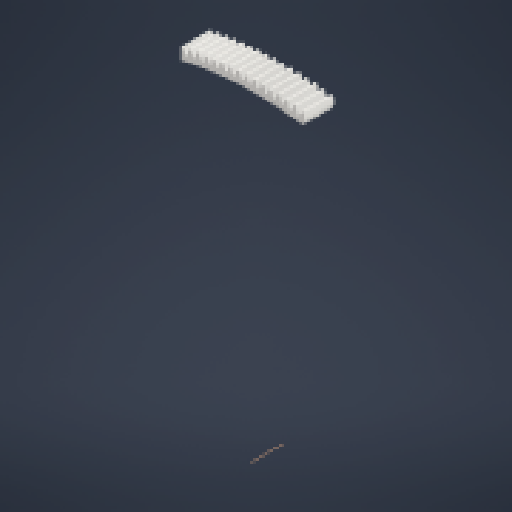
# Autodesk Inventor part: Цилиндрическое зубчатое зацепление2
Saved by Autodesk Inventor 2026.2 (Build 302298000, 298)
## iProperties
CustomPartVersion: 1
Created: 2025-12-07
Part Number: Цилиндрическое зубчатое зацепление2
Material: Steel
Document SubType Name: Modeling
Designer: Phantom
Categories: <?xml version="1.0" encoding="UTF-16"?> <MemberInstance><Categories><FamilyTemplate><FamilyTemplateParameter ValueType="xs:double" Id="1" ObjectReferenceKey="da_z" ObjectType="kUserParameterObject"/><FamilyTemplateParameter ValueType="xs:double" Id="2" ObjectReferenceKey="da_b" ObjectType="kUserParameterObject"/><FamilyTemplateParameter ValueType="xs:double" Id="3" ObjectReferenceKey="da_beta" ObjectType="kUserParameterObject"/><FamilyTemplateParameter ValueType="xs:double" Id="4" ObjectReferenceKey="da_da" ObjectType="kUserParameterObject"/><FamilyTemplateParameter ValueType="xs:double" Id="5" ObjectReferenceKey="da_aw" ObjectType="kUserParameterObject"/><FamilyTemplateParameter ValueType="xs:string" Id="6" ObjectReferenceKey="EAIAABAAAACIAQAAAAAAAIAAAAAAAAAA" ObjectType="83910656" SubObjectId="SurfaceGeometry"/></FamilyTemplate><ParamToTemplateMap><ParamToTemplate CategoryParameter="//CategoryParameter[@InternalName='046C89C9-8512-4d59-83FE-43B91F4F132A']" TemplateParameter="1"/><ParamToTemplate CategoryParameter="//CategoryParameter[@InternalName='2552DF32-E462-4b46-AEBF-C6C7768E72AC']" TemplateParameter="2"/><ParamToTemplate CategoryParameter="//CategoryParameter[@InternalName='C9EE641D-15FC-4fae-A226-E94C4372FDD7']" TemplateParameter="3"/><ParamToTemplate><ParamToTemplate CategoryParameter="//CategoryParameter[@InternalName='00B6519A-459B-49c7-AD84-2E56D39A5744']" ConstantValue="0.580360"/></ParamToTemplate><ParamToTemplate><ParamToTemplate CategoryParameter="//CategoryParameter[@InternalName='04B31F0E-C7A6-4894-AA32-9629BEFACF47']" ConstantValue="1.000000"/></ParamToTemplate><ParamToTemplate><ParamToTemplate CategoryParameter="//CategoryParameter[@InternalName='43CBEC2E-7847-49e7-A936-2F7889FCB2D9']" ConstantValue="0.250000"/></ParamToTemplate><ParamToTemplate><ParamToTemplate CategoryParameter="//CategoryParameter[@InternalName='B1EFC894-105D-4ebd-86BF-FA20ED196853']" ConstantValue="0.350000"/></ParamToTemplate><ParamToTemplate><ParamToTemplate CategoryParameter="//CategoryParameter[@InternalName='51175063-3D10-4879-93E8-6246FE8B403D']" ConstantValue="2060000000.000000"/></ParamToTemplate><ParamToTemplate><ParamToTemplate CategoryParameter="//CategoryParameter[@InternalName='A3A52E27-4454-46a9-B0BD-C932399B70AF']" ConstantValue="0.300000"/></ParamToTemplate><ParamToTemplate><ParamToTemplate CategoryParameter="//CategoryParameter[@InternalName='91B76062-C214-41d9-B1B9-14D2AB99603D']" ConstantValue="0.175000"/></ParamToTemplate><ParamToTemplate><ParamToTemplate CategoryParameter="//CategoryParameter[@InternalName='374E806E-8B8A-4dda-A9AA-1039D6500AD2']" ConstantValue="5.714286"/></ParamToTemplate><ParamToTemplate><ParamToTemplate CategoryParameter="//CategoryParameter[@InternalName='2D373A89-B862-43d6-8D0B-0CBF12AB9F6C']" ConstantValue="0.349066"/></ParamToTemplate><ParamToTemplate CategoryParameter="//CategoryParameter[@InternalName='37777632-D6A2-4fac-9D53-DB8ACD95C989']" TemplateParameter="4"/><ParamToTemplate CategoryParameter="//CategoryParameter[@InternalName='FD1017F1-B727-4f7e-9707-0F86F1FF9423']" TemplateParameter="5"/><ParamToTemplate><ParamToTemplate CategoryParameter="//CategoryParameter[@InternalName='9E1B4470-B2D3-4ff1-B813-535BB4CDF51A']" ConstantValue="3520000.000000"/></ParamToTemplate><ParamToTemplate><ParamToTemplate CategoryParameter="//CategoryParameter[@InternalName='F8452263-BFF6-458c-9FB1-07C4B99E95CD']" ConstantValue="11400000.000000"/></ParamToTemplate><ParamToTemplate><ParamToTemplate CategoryParameter="//CategoryParameter[@InternalName='3E3BB259-FD49-497f-8171-6EBC954A3479']" ConstantValue="2.000000"/></ParamToTemplate><ParamToTemplate CategoryParameter="//CategoryParameter[@InternalName='27C3BAF2-7550-4e4b-AE2C-0DB134B7D9B7']" TemplateParameter="6"/></ParamToTemplateMap><Category DisplayName="Gear" InternalName="DC85795E-93AB-48d5-8EEE-5A27447B64BD" Mnemonic="Gear"><CategoryParameter DisplayName="z" InternalName="046C89C9-8512-4d59-83FE-43B91F4F132A" Mnemonic="z"/><CategoryParameter DisplayName="b" InternalName="2552DF32-E462-4b46-AEBF-C6C7768E72AC" Mnemonic="b"/><CategoryParameter DisplayName="||b|" InternalName="C9EE641D-15FC-4fae-A226-E94C4372FDD7" Mnemonic="beta"/><CategoryParameter DisplayName="x" InternalName="00B6519A-459B-49c7-AD84-2E56D39A5744" Mnemonic="x"/><CategoryParameter DisplayName="a*" InternalName="04B31F0E-C7A6-4894-AA32-9629BEFACF47" Mnemonic="a"/><CategoryParameter DisplayName="c*" InternalName="43CBEC2E-7847-49e7-A936-2F7889FCB2D9" Mnemonic="c"/><CategoryParameter DisplayName="r|.f|*" InternalName="B1EFC894-105D-4ebd-86BF-FA20ED196853" Mnemonic="rf"/><CategoryParameter DisplayName="E" InternalName="51175063-3D10-4879-93E8-6246FE8B403D" Mnemonic="E"/><CategoryParameter DisplayName="||m|" InternalName="A3A52E27-4454-46a9-B0BD-C932399B70AF" Mnemonic="mi"/><Category DisplayName="SpurGear" InternalName="26C5A22E-A91E-4dfd-A3B3-23CCAFAE1764" Mnemonic="SpurGear"><CategoryParameter DisplayName="m" InternalName="91B76062-C214-41d9-B1B9-14D2AB99603D" Mnemonic="m"/><CategoryParameter DisplayName="P" InternalName="374E806E-8B8A-4dda-A9AA-1039D6500AD2" Mnemonic="PP"/><CategoryParameter DisplayName="||a|" InternalName="2D373A89-B862-43d6-8D0B-0CBF12AB9F6C" Mnemonic="alpha"/><CategoryParameter DisplayName="d|.a|" InternalName="37777632-D6A2-4fac-9D53-DB8ACD95C989" Mnemonic="da"/><CategoryParameter DisplayName="a|.w|" InternalName="FD1017F1-B727-4f7e-9707-0F86F1FF9423" Mnemonic="aw"/><CategoryParameter DisplayName="||s||.Flim|" InternalName="9E1B4470-B2D3-4ff1-B813-535BB4CDF51A" Mnemonic="sFlim"/><CategoryParameter DisplayName="||s||.Hlim|" InternalName="F8452263-BFF6-458c-9FB1-07C4B99E95CD" Mnemonic="sHlim"/><CategoryParameter DisplayName="тип" InternalName="3E3BB259-FD49-497f-8171-6EBC954A3479" Mnemonic="type"/><CategoryParameter DisplayName="PitchDiameter" InternalName="27C3BAF2-7550-4e4b-AE2C-0DB134B7D9B7" Mnemonic="IDS_PITCHDIAM"/></Category></Category></Categories></MemberInstance>
Density: 1 g/cm^3
Appearance: Steel
Author: Phantom
Autodesk Inventor part; units mm, degrees
sketch "Sketch1" plane through (0, 0, 0) normal (0, 0, 1) x (1, 0, 0)
  circle A0 centre (0, 0) radius 225.875
  dimension "d0" = 451.75
  constraints: 1 centre point
  measures "d0" diameter of A0
extrude "Extrusion1" add sketch "Sketch1" along normal blind 20
ref_plane "Work Plane2" through (0, 0, 10) normal (0, 0, 1) x (1, 0, 0)
sketch "Sketch2" plane through (0, 0, 0) normal (0, 0, -1) x (-1, 0, 0)
  circle A0 centre (0, 0) radius 225.875 projected
  circle A1 centre (0, 0) radius 223.125
  dimension "d3" = 446.25
  constraints: 1 centre point, 1 coincident
  measures "d3" diameter of A1
surface extrude "Средний диаметр" sketch "Sketch2" against normal through all shown no curves A1
ref_plane "Work Plane8" through (0, 0, 0) normal (0.9999241, 0.0123197, 0) x (0, 0, 1)
ref_plane "Work Plane9" through (0, 0, 0) normal (1, 0, 0) x (0, 1, 0)
spur gear teeth "Цилиндрическое зубчатое зацепление" teeth 255 pitch diameter 446.25 tip diameter 451.75 root diameter 443.9063 face width 20 start plane through (0, 0, 0) normal (0, 0, -1) x (-1, 0, 0)
sketch "Эскиз3" plane through (0, 0, 20) normal (0, 0, 1) x (1, 0, 0)
  line L0 (-50.0802, 214.6531) -> (-50.0464, 212.2194) projected
  line L1 (35.7305, 217.5025) -> (34.832, 215.2404) projected
  line L2 (-50.0802, 214.6531) -> (-50.0802, 276.5241)
  line L3 (34.832, 215.2404) -> (59.7862, 278.0604)
  line L4 (35.7305, 217.5025) -> (36.2471, 218.803) projected
  circle A0 centre (0, 0) radius 218.0406
  circle A1 centre (0, 0) radius 281.0224
  point P0 (58.5159, 274.8626)
  constraints: 4 end point, 2 coincident, 1 collinear, 1 vertical, 6 other
extrude "Выдавливание2" cut sketch "Эскиз3" against normal through all contours L0 A0 L1 L3 A1 L2 | A0 picked at (-244.7051, -87.2795)
sketch "Эскиз4" plane through (0, 0, 0) normal (0, 0, -1) x (-1, 0, 0)
  line L0 (50.0802, 214.6531) -> (50.0802, 220.2532) projected
  arc A0 (50.0802, 220.2532) -> (49.0015, 220.4957) centre (0, 0) ccw projected
  arc A1 (49.0015, 220.4957) -> (46.8151, 216.9598) centre (71.1043, 204.3851) ccw projected
  arc A2 (46.8151, 216.9598) -> (45.4778, 217.244) centre (0, 0) ccw projected
  arc A3 (45.4778, 217.244) -> (44.9186, 221.3636) centre (18.1739, 215.6358) ccw projected
  arc A4 (44.9186, 221.3636) -> (43.5542, 221.6361) centre (0, 0) ccw projected
  arc A5 (43.5542, 221.6361) -> (41.4556, 218.0473) centre (66.0472, 206.0749) ccw projected
  arc A6 (41.4556, 218.0473) -> (40.1116, 218.2985) centre (0, 0) ccw projected
  arc A7 (40.1116, 218.2985) -> (39.4511, 222.4031) centre (12.8557, 216.0181) ccw projected
  arc A8 (39.4511, 222.4031) -> (38.0804, 222.6419) centre (0, 0) ccw projected
  arc A9 (38.0804, 222.6419) -> (36.0708, 219.0025) centre (60.95, 207.6395) ccw projected
  arc A10 (36.0708, 219.0025) -> (34.7211, 219.2205) centre (0, 0) ccw projected
  arc A11 (34.7211, 219.2205) -> (33.9597, 223.3075) centre (7.5296, 216.2692) ccw projected
  arc A12 (33.9597, 223.3075) -> (32.5835, 223.5125) centre (0, 0) ccw projected
  arc A13 (32.5835, 223.5125) -> (30.6642, 219.8247) centre (55.8158, 209.0782) ccw projected
  arc A14 (30.6642, 219.8247) -> (29.3095, 220.0094) centre (0, 0) ccw projected
  arc A15 (29.3095, 220.0094) -> (28.4477, 224.0764) centre (2.199, 216.3891) ccw projected
  arc A16 (28.4477, 224.0764) -> (27.0668, 224.2474) centre (0, 0) ccw projected
  arc A17 (27.0668, 224.2474) -> (25.239, 220.5135) centre (50.6477, 210.3899) ccw projected
  arc A18 (25.239, 220.5135) -> (23.8802, 220.6647) centre (0, 0) ccw projected
  arc A19 (23.8802, 220.6647) -> (22.9184, 224.7093) centre (-3.1329, 216.3776) ccw projected
  arc A20 (22.9184, 224.7093) -> (21.5337, 224.8462) centre (0, 0) ccw projected
  arc A21 (21.5337, 224.8462) -> (19.7985, 221.0683) centre (45.4488, 211.5738) ccw projected
  arc A22 (19.7985, 221.0683) -> (18.4363, 221.1861) centre (0, 0) ccw projected
  arc A23 (18.4363, 221.1861) -> (17.3752, 225.2057) centre (-8.463, 216.2347) ccw projected
  arc A24 (17.3752, 225.2057) -> (15.9876, 225.3085) centre (0, 0) ccw projected
  arc A25 (15.9876, 225.3085) -> (14.3459, 221.489) centre (40.2224, 212.6293) ccw projected
  arc A26 (14.3459, 221.489) -> (12.9813, 221.5732) centre (0, 0) ccw projected
  arc A27 (12.9813, 221.5732) -> (11.8214, 225.5654) centre (-13.7879, 215.9606) ccw projected
  arc A28 (11.8214, 225.5654) -> (10.4317, 225.634) centre (0, 0) ccw projected
  arc A29 (10.4317, 225.634) -> (8.8846, 221.7752) centre (34.9715, 213.5558) ccw projected
  arc A30 (8.8846, 221.7752) -> (7.5183, 221.8258) centre (0, 0) ccw projected
  arc A31 (7.5183, 221.8258) -> (6.2604, 225.7882) centre (-19.1044, 215.5553) ccw projected
  arc A32 (6.2604, 225.7882) -> (4.8695, 225.8225) centre (0, 0) ccw projected
  arc A33 (4.8695, 225.8225) -> (3.4179, 221.9268) centre (29.6994, 214.3526) ccw projected
  arc A34 (3.4179, 221.9268) -> (2.0508, 221.9437) centre (0, 0) ccw projected
  arc A35 (2.0508, 221.9437) -> (0.6957, 225.8739) centre (-24.4093, 215.0192) ccw projected
  arc A36 (0.6957, 225.8739) -> (-0.6957, 225.8739) centre (0, 0) ccw projected
  arc A37 (-0.6957, 225.8739) -> (-2.0508, 221.9437) centre (24.4093, 215.0192) ccw projected
  arc A38 (-2.0508, 221.9437) -> (-3.4179, 221.9268) centre (0, 0) ccw projected
  arc A39 (-3.4179, 221.9268) -> (-4.8695, 225.8225) centre (-29.6994, 214.3526) ccw projected
  arc A40 (-4.8695, 225.8225) -> (-6.2604, 225.7882) centre (0, 0) ccw projected
  arc A41 (-6.2604, 225.7882) -> (-7.5183, 221.8258) centre (19.1044, 215.5553) ccw projected
  arc A42 (-7.5183, 221.8258) -> (-8.8846, 221.7752) centre (0, 0) ccw projected
  arc A43 (-8.8846, 221.7752) -> (-10.4317, 225.634) centre (-34.9715, 213.5558) ccw projected
  arc A44 (-10.4317, 225.634) -> (-11.8214, 225.5654) centre (0, 0) ccw projected
  arc A45 (-11.8214, 225.5654) -> (-12.9813, 221.5732) centre (13.7879, 215.9606) ccw projected
  arc A46 (-12.9813, 221.5732) -> (-14.3459, 221.489) centre (0, 0) ccw projected
  arc A47 (-14.3459, 221.489) -> (-15.9876, 225.3085) centre (-40.2224, 212.6293) ccw projected
  arc A48 (-15.9876, 225.3085) -> (-17.3752, 225.2057) centre (0, 0) ccw projected
  arc A49 (-17.3752, 225.2057) -> (-18.4363, 221.1861) centre (8.463, 216.2347) ccw projected
  arc A50 (-18.4363, 221.1861) -> (-19.7985, 221.0683) centre (0, 0) ccw projected
  arc A51 (-19.7985, 221.0683) -> (-21.5337, 224.8462) centre (-45.4488, 211.5738) ccw projected
  arc A52 (-21.5337, 224.8462) -> (-22.9184, 224.7093) centre (0, 0) ccw projected
  arc A53 (-22.9184, 224.7093) -> (-23.8802, 220.6647) centre (3.1329, 216.3776) ccw projected
  arc A54 (-23.8802, 220.6647) -> (-25.239, 220.5135) centre (0, 0) ccw projected
  arc A55 (-25.239, 220.5135) -> (-27.0668, 224.2474) centre (-50.6477, 210.3899) ccw projected
  arc A56 (-27.0668, 224.2474) -> (-28.4477, 224.0764) centre (0, 0) ccw projected
  arc A57 (-28.4477, 224.0764) -> (-29.3095, 220.0094) centre (-2.199, 216.3891) ccw projected
  arc A58 (-29.3095, 220.0094) -> (-30.6642, 219.8247) centre (0, 0) ccw projected
  arc A59 (-30.6642, 219.8247) -> (-32.5835, 223.5125) centre (-55.8158, 209.0782) ccw projected
  arc A60 (-32.5835, 223.5125) -> (-33.9597, 223.3075) centre (0, 0) ccw projected
  arc A61 (-33.9597, 223.3075) -> (-34.7211, 219.2205) centre (-7.5296, 216.2692) ccw projected
  arc A62 (-34.7211, 219.2205) -> (-36.0708, 219.0025) centre (0, 0) ccw projected
  arc A63 (-36.0708, 219.0025) -> (-37.2044, 221.2129) centre (-60.95, 207.6395) ccw projected
  line L1 (-37.2044, 221.2129) -> (-34.832, 215.2404) projected
  arc A64 (50.0464, 212.2194) -> (-34.832, 215.2404) centre (0, 0) ccw projected
  line L2 (50.0464, 212.2194) -> (50.0802, 214.6531) projected
  line L3 (-34.1401, 217.7578) -> (-33.24, 215.492) projected
  line L4 (-33.24, 215.492) -> (-35.2347, 220.5135)
  point P0 (-34.7211, 219.2205)
  constraints: 2 end point
extrude "Выдавливание3" cut sketch "Эскиз4" against normal through all contours A64 L1 A63 A62 L4 L3
equation "\"d0\" = da_da"
equation "\"d1\" = da_b"
equation "\"d3\" = da_d"
equation "\"d16\" = da_aw"
equation "\"d43\" = da_aw"
equation "\"d46\" = da_aw"
equation "\"da_da\" = 451.75"
equation "\"da_b\" = 20"
equation "\"da_d\" = 446.25"
equation "\"da_aw\" = 239"
body "Solid1"
body "Srf1"
